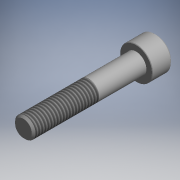
# Autodesk Inventor part: DIN-912 - M10x55(F)
Saved by Autodesk Inventor 2017.3 (Build 213256000, 256)
## iProperties
Part Number: DIN-912 - M10x55(F)
Material: Generic
Catalog Web Link: www.cadenas.de
Description: DIN-912-Cylinder screw
Vendor: FESTO
Document SubType Name: Modeling
Designer: partserver
Manufacturer: FESTO
Mass: 5.97434 g
Surface Area: 27.1493 cm^2
Volume: 5.97434 cm^3
Density: 1 g/cm^3
Appearance: PSOLRGB-192-192-192
Category: PARTsolutions
Company: FESTO
Title: DIN-912 - M10x55(F)
Author: Cadenas PARTsolutions
Comments: Cylinder screw
PSOL_IDENT_0: {$CADENAS_DATA\23d-libs\festo\zyl_zubeh\d912\din_912.prj},180 {VTYP=3D},{NB=DIN-912 - M10x55(F)},{LI
PSOL_IDENT_1: NA=DIN-912 - M10x55(F)},{NN=DIN-912},{DATE=01.07.2020 05:33:41},{GEOMDATE=01.07.2020 05:33:34},{VERS
PSOL_IDENT_2: ION=},{LINEID=790},{WBVAR=},{WBNUMERIC=}  {NB=DIN-912 - M10x55(F)},{LINA=DIN-912 - M10x55(F)},{KT=X}
PSOL_IDENT_3: ,{IDNR=},{GEW=M10},{DG=10.000},{P=1.500},{L=55.000},{B=32.000},{FORM=0},{GKD=8.160},{DK=16.000},{DAD
PSOL_IDENT_4: IN=11.200},{DS=10.000},{E=9.150},{LF=1.020},{K=10.000},{R=0.400},{S=8.000},{T=5.000},{V=1.000},{DW=1
PSOL_IDENT_5: 5.330},{W=4.000},{NENN=M10x55},{DA=10.1},{BL=32}
NB: DIN-912 - M10x55(F)
NN: DIN-912
NT: Cylinder screw
NBSYN: DIN-912 - $NENN.(F)
LINA: DIN-912 - M10x55(F)
CATALOG: Festo
ROWDESC: M10x55
GEW: M10
DG: 10
P: 1.5
L: 55
B: 32
FORM: 0
GKD: 8.16
DK: 16
DADIN: 11.2
DS: 10
E: 9.15
LF: 1.02
K: 10
R: 0.4
S: 8
T: 5
V: 1
DW: 15.33
W: 4
SUPPLIER: FESTO
ARTICLENO: DIN-912 - M10x55(F)
BOMINFO: DIN-912 - M10x55(F)
CREATOR: CADENAS GmbH
Autodesk Inventor part; units mm, degrees
sketch "Sketch_1" plane through (0, 0, 0) normal (0, 0, 1) x (1, 0, 0)
  line L0 (0, -55) -> (0, 10)
  line L1 (0, 2.6906) -> (4, 5)
  line L2 (4, 5) -> (4, 9.3812)
  line L3 (4, 9.3812) -> (4.6188, 10)
  line L4 (4.6188, 10) -> (7, 10)
  line L5 (7, 10) -> (8, 9)
  line L6 (8, 9) -> (8, 0.25)
  line L7 (8, 0.25) -> (7.75, 0)
  line L8 (7.75, 0) -> (5.05, 0)
  line L9 (5.05, 0) -> (5, -1.02)
  line L10 (5, -1.02) -> (5, -54.08)
  line L11 (5, -54.08) -> (4.08, -55)
  line L12 (4.08, -55) -> (0, -55)
  line L13 (0, -55) -> (0, 2.6906)
  constraints: 28 end point
revolve "Revolution1" add sketch "Sketch_1" angle 360 about axis through (0, -55, 0) along (0, -1, 0)
thread "Thread1" size "M10x1.5" class "6g" standard "ISO Metric profile" length 31.08
sketch "Sketch_2" plane through (0, 10, 0) normal (0, 1, 0) x (1, 0, 0)
  line L0 (-4, -2.3094) -> (0, -4.6188)
  line L1 (0, -4.6188) -> (4, -2.3094)
  line L2 (4, -2.3094) -> (4, 2.3094)
  line L3 (4, 2.3094) -> (0, 4.6188)
  line L4 (0, 4.6188) -> (-4, 2.3094)
  line L5 (-4, 2.3094) -> (-4, -2.3094)
  constraints: 12 end point
extrude "Extrusion1" cut sketch "Sketch_2" against normal blind 5
ref_plane "ANBAU_XY" through (0, 0, 0) normal (0, 1, 0) x (1, 0, 0)
ref_plane "ANBAU_YZ" through (0, 0, 0) normal (1, 0, 0) x (0, 0, -1)
ref_plane "ANBAU_ZX" through (0, 0, 0) normal (0, 0, -1) x (0, 1, 0)
ref_plane "Schraube_XY" through (0, 0, 0) normal (0, 1, 0) x (1, 0, 0)
ref_plane "Schraube_YZ" through (0, 0, 0) normal (1, 0, 0) x (0, 0, -1)
ref_plane "Schraube_ZX" through (0, 0, 0) normal (0, 0, -1) x (0, 1, 0)
ref_plane "insert_XY" through (0, 0, 0) normal (0, 1, 0) x (1, 0, 0)
ref_plane "insert_YZ" through (0, 0, 0) normal (1, 0, 0) x (0, 0, -1)
ref_plane "insert_ZX" through (0, 0, 0) normal (0, 0, -1) x (0, 1, 0)
ref_plane "schrauben_punkt_XY" through (0, -55, 0) normal (0, 1, 0) x (1, 0, 0)
ref_plane "schrauben_punkt_YZ" through (0, -55, 0) normal (1, 0, 0) x (0, 0, -1)
ref_plane "schrauben_punkt_ZX" through (0, -55, 0) normal (0, 0, -1) x (0, 1, 0)
body "Solid1"
